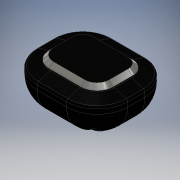
# Autodesk Inventor part: camera
Saved by Autodesk Inventor 2016 (Build 200138000, 138)
## iProperties
Created: 2016-03-19
Part Number: camera
Material: Generic
Document SubType Name: Modeling
Designer: Hamid Osooli
Density: 1 g/cm^3
Appearance: Anodized - Black
Mass: 23.0823 g
Surface Area: 51.0944 cm^2
Volume: 23.0823 cm^3
Author: Hamid Osooli
Autodesk Inventor part; units mm, degrees
ref_plane "YZ Plane" through (0, 0, 0) normal (1, 0, 0) x (0, 1, 0)
ref_plane "XZ Plane" through (0, 0, 0) normal (0, 1, 0) x (-1, 0, 0)
sketch "Sketch1" plane through (0, 0, 0) normal (0, 0, 1) x (1, 0, 0)
  line L0 (-7.25, -17.75) -> (7.25, -17.75)
  line L1 (22.25, -2.75) -> (22.25, 5.75)
  line L2 (8.25, 19.75) -> (-8.25, 19.75)
  line L3 (-22.25, 5.75) -> (-22.25, -2.75)
  line L4 (-23.8636, 0) -> (23.8636, 0)
  arc A0 (-8.25, 19.75) -> (-22.25, 5.75) centre (-8.25, 5.75) ccw
  arc A1 (22.25, 5.75) -> (8.25, 19.75) centre (8.25, 5.75) ccw
  arc A2 (-22.25, -2.75) -> (-7.25, -17.75) centre (-7.25, -2.75) ccw
  arc A3 (7.25, -17.75) -> (22.25, -2.75) centre (7.25, -2.75) ccw
  line L5 (-8.7303, 13.1919) -> (8.6193, 13.1919)
  line L6 (15.6193, 6.1919) -> (15.6193, -3.1827)
  line L7 (7.6193, -11.1827) -> (-7.7303, -11.1827)
  line L8 (-15.7303, -3.1827) -> (-15.7303, 6.1919)
  arc A4 (15.6193, 6.1919) -> (8.6193, 13.1919) centre (8.6193, 6.1919) ccw
  arc A5 (7.6193, -11.1827) -> (15.6193, -3.1827) centre (7.6193, -3.1827) ccw
  arc A6 (-8.7303, 13.1919) -> (-15.7303, 6.1919) centre (-8.7303, 6.1919) ccw
  arc A7 (-15.7303, -3.1827) -> (-7.7303, -11.1827) centre (-7.7303, -3.1827) ccw
  point P0 (0, 0)
  point P1 (-22.25, -17.75)
  point P2 (22.25, -17.75)
  point P3 (22.25, 19.75)
  point P4 (-22.25, 19.75)
  point P5 (-22.25, 19.75)
  point P6 (-22.25, 19.75)
  point P7 (-22.25, 19.75)
  point P8 (22.25, 19.75)
  point P9 (22.25, 19.75)
  point P10 (22.25, 19.75)
  point P11 (-22.25, -17.75)
  point P12 (-22.25, -17.75)
  point P13 (-22.25, -17.75)
  point P14 (22.25, -17.75)
  point P15 (22.25, -17.75)
  point P16 (22.25, -17.75)
  point P17 (0, 0)
  dimension "d51" = 0
  dimension "d52" = 0
  dimension "d0" = 44.5
  dimension "d1" = 37.5
  dimension "d2" = 44.5
  dimension "d283" = 14
  dimension "d284" = 14
  dimension "d285" = 15
  dimension "d286" = 15
  dimension "d293" = 7
  dimension "d295" = 8
  dimension "d299" = 7
  dimension "d300" = 8
  constraints: 18 end point, 16 point on circle, 16 point on line, 16 tangent, 8 centre point, 6 horizontal, 4 vertical, 3 perpendicular, 2 parallel, 1 coincident, 1 midpoint, 16 other
  measures "d0" distance of point (-22.25, -17.75) point (22.25, -17.75)
  measures "d1" distance of point (22.25, -17.75) point (22.25, 19.75)
  measures "d2" distance of point (22.25, 19.75) point (-22.25, 19.75)
  measures "d283" radius of A0
  measures "d284" radius of A1
  measures "d285" radius of A2
  measures "d286" radius of A3
  measures "d293" radius of A4
  measures "d295" radius of A5
  measures "d299" radius of A6
  measures "d300" radius of A7
extrude "Extrusion1" add sketch "Sketch1" against normal blind 19
sketch "Sketch3" plane through (0, 0, -19) normal (0, 0, -1) x (-1, 0, 0)
  line L0 (-22.25, 5.75) -> (-22.25, -2.75) projected
  line L1 (22.25, -2.75) -> (22.25, 5.75) projected
  line L2 (-15.5, -8.0593) -> (15.5, -8.0593)
  line L3 (15.5, -8.0593) -> (15.5, -12.5593)
  line L4 (15.5, -12.5593) -> (-15.5, -12.5593)
  line L5 (-15.5, -12.5593) -> (-15.5, -8.0593)
  point P0 (0, 0)
  point P1 (-22.25, 19.75)
  point P2 (-22.25, -17.75)
  point P3 (22.25, -17.75)
  point P4 (22.25, 19.75)
  dimension "d269" = 31
  constraints: 8 end point, 1 perpendicular
  measures "d269" distance of L2.start L2.end
extrude "Extrusion2" cut sketch "Sketch3" against normal blind 10
fillet "Fillet1" radius 14 1 edges at (0, 19.75, -19)
chamfer "Chamfer1" distance 2 angle 73 1 edges at (0, 19.75, 0) measured on face at (2.75, 19.75, -1.6667)
fillet "Fillet3" radius 1 1 edges at (0, 19.75, -2)
extrude "Extrusion4" add sketch "Sketch1" along normal blind 2.5 contours L8 A6 L5 A4 L6 L4 | L4 L6 A5 L7 A7 L8
chamfer "Chamfer4" distance 2 angle 45 8 edges at (-0.0555, 13.1919, 2.5) (-13.68, 11.1417, 2.5) (-15.7303, 1.5046, 2.5) (-13.3871, -8.8395, 2.5) (-0.0555, -11.1827, 2.5) (13.2762, -8.8395, 2.5) (15.6193, 1.5046, 2.5) (13.5691, 11.1417, 2.5) measured on face at (-2.6137, 5.0671, 2.5)
ref_plane "Work Plane4" through (-8.25, -0.7605, -19) normal (0, 0, -1) x (-1, 0, 0)
sketch "Sketch4" plane through (-8.25, -0.7605, -19) normal (0, 0, -1) x (-1, 0, 0)
  circle A0 centre (-8.25, 1.7719) radius 4.5
  point P0 (-8.25, 0.7605)
  dimension "d313" = 9
  constraints: 1 centre point
  measures "d313" diameter of A0
extrude "Extrusion5" add sketch "Sketch4" along normal blind 5 draft -30
body "Solid1"
